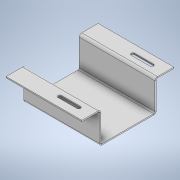
# Autodesk Inventor part: CameraProtection
Saved by Autodesk Inventor 2020 (Build 240168000, 168)
## iProperties
Created: 2019-11-07
Part Number: CameraProtection
Material: Generic
Document SubType Name: Sheet Metal
Designer: nicoc
Density: 1 g/cm^3
Sheet Metal Rule: Default_mm
Appearance: Default
Author: nicoc
Autodesk Inventor part; units mm, degrees
ref_plane "YZ Plane" through (0, 0, 0) normal (1, 0, 0) x (0, 1, 0)
ref_plane "XZ Plane" through (0, 0, 0) normal (0, 1, 0) x (-1, 0, 0)
ref_plane "XY Plane" through (0, 0, 0) normal (0, 0, 1) x (1, 0, 0)
sketch "Sketch1" plane through (0, 0, 0) normal (0, 1, 0) x (-1, 0, 0)
  line L0 (0, 0) -> (120, 0)
  line L1 (120, 0) -> (120, -30)
  line L2 (120, -30) -> (0, -30)
  line L3 (0, -30) -> (0, 0)
  dimension "d41" = 120
  dimension "d42" = 30
  measures "d41" distance between parallel lines of L1 L3
  measures "d42" distance between parallel lines of L0 L2
extrude "Plate1" add sketch "Sketch1" along normal mid plane 2
sketch "Sketch6" plane through (0, 1, -28) normal (0, 0, -1) x (-1, 0, 0)
  line L0 (120, 0) -> (0, 0)
  line L1 (0, 0) -> (0, -50)
  line L2 (0, -50) -> (120, -50)
  line L3 (120, -50) -> (120, 0)
  constraints: 6 end point, 1 horizontal, 1 perpendicular, 1 vertical
edge flange "Flange5" height 50 angle 90 thickness 2 bend radius 2 thickness toward (0, 0, -1) relief tear relief width 2 relief depth 1 edges at (-60, -1, -30) wall of the first edge with corners at (-120, 1, -28) (0, 1, -28) (0, -49, -28) (-120, -49, -28)
bend "Bend5"
corner "Corner5"
sketch "Sketch7" plane through (-120, -47, -28) normal (0, -1, 0) x (1, 0, 0)
  line L0 (120, 0) -> (0, 0)
  line L1 (0, 0) -> (0, -90)
  line L2 (0, -90) -> (120, -90)
  line L3 (120, -90) -> (120, 0)
  constraints: 6 end point, 1 horizontal, 1 perpendicular, 1 vertical
edge flange "Flange6" height 90 angle 90 thickness 2 bend radius 2 thickness toward (0, -1, 0) relief tear relief width 2 relief depth 1 edges at (-60, -49, -30) wall of the first edge with corners at (0, -47, -28) (-120, -47, -28) (-120, -47, -118) (0, -47, -118)
bend "Bend6"
corner "Corner6"
sketch "Sketch8" plane through (-120, -49, -116) normal (0, 0, -1) x (-1, 0, 0)
  line L0 (-120, 0) -> (0, 0)
  line L1 (0, 0) -> (0, 50)
  line L2 (0, 50) -> (-120, 50)
  line L3 (-120, 50) -> (-120, 0)
  constraints: 6 end point, 1 horizontal, 1 perpendicular, 1 vertical
edge flange "Flange7" height 50 angle 90 thickness 2 bend radius 2 thickness toward (0, 0, -1) relief tear relief width 2 relief depth 1 edges at (-60, -47, -118) wall of the first edge with corners at (0, -49, -116) (-120, -49, -116) (-120, 1, -116) (0, 1, -116)
bend "Bend7"
corner "Corner7"
sketch "Sketch9" plane through (0, -1, -116) normal (0, 1, 0) x (-1, 0, 0)
  line L0 (120, 0) -> (0, 0)
  line L1 (0, 0) -> (0, -30)
  line L2 (0, -30) -> (120, -30)
  line L3 (120, -30) -> (120, 0)
  constraints: 6 end point, 1 horizontal, 1 perpendicular, 1 vertical
edge flange "Flange8" height 30 angle 90 thickness 2 bend radius 2 thickness toward (0, 1, 0) relief tear relief width 2 relief depth 1 edges at (-60, 1, -118) wall of the first edge with corners at (-120, -1, -116) (0, -1, -116) (0, -1, -146) (-120, -1, -146)
bend "Bend8"
corner "Corner8"
sketch "Sketch15" plane through (0, -1, 0) normal (0, -1, 0) x (1, 0, 0)
  line L0 (-17.25, -15) -> (-52.75, -15) construction
  line L1 (-20, -17.75) -> (-50, -17.75)
  line L2 (-50, -12.25) -> (-20, -12.25)
  arc A0 (-20, -17.75) -> (-20, -12.25) centre (-20, -15) ccw
  arc A1 (-50, -12.25) -> (-50, -17.75) centre (-50, -15) ccw
  line L3 (0, -26) -> (0, 0) projected
  line L4 (0, 0) -> (-120, 0) projected
  point P0 (-35, -15)
  dimension "d130" = 20
  dimension "d131" = 15
  dimension "d132" = 30
  dimension "d133" = 5.5
  constraints: 8 end point, 6 point on circle, 4 tangent, 2 centre point, 2 point on line, 1 horizontal, 1 midpoint, 1 parallel
  measures "d130" distance from line of L3 A0.centre
  measures "d131" distance from line of L4 A0.centre
  measures "d132" distance of A1.centre A0.centre
  measures "d133" distance between parallel lines of L1 L2
extrude "Cut3" cut sketch "Sketch15" against normal blind 2
sketch "Sketch16" plane through (-120, -1, -146) normal (0, -1, 0) x (1, 0, 0)
  line L0 (102.75, 15) -> (67.25, 15) construction
  line L1 (100, 17.75) -> (70, 17.75)
  line L2 (70, 12.25) -> (100, 12.25)
  arc A0 (100, 12.25) -> (100, 17.75) centre (100, 15) ccw
  arc A1 (70, 17.75) -> (70, 12.25) centre (70, 15) ccw
  line L3 (120, 26) -> (120, 0) projected
  line L4 (0, 0) -> (120, 0) projected
  point P0 (120, 146)
  point P1 (85, 15)
  dimension "d136" = 20
  dimension "d137" = 15
  dimension "d138" = 5.5
  dimension "d139" = 30
  constraints: 8 end point, 6 point on circle, 4 tangent, 2 centre point, 2 point on line, 1 horizontal, 1 midpoint, 1 parallel
  measures "d136" distance from line of L3 A0.centre
  measures "d137" distance from line of L4 A0.centre
  measures "d138" distance between parallel lines of L2 L1
  measures "d139" distance of A1.centre A0.centre
extrude "Cut4" cut sketch "Sketch16" against normal blind 2
equation "\"d134\" = Thickness"
equation "\"d140\" = Thickness"
equation "\"d0\" = Thickness"
equation "\"d43\" = BendReliefWidth"
equation "\"d44\" = BendReliefDepth"
equation "\"d45\" = MinimumRemnant"
equation "\"d46\" = TransitionRadius"
equation "\"d49\" = BendRadius"
equation "\"d50\" = CornerReliefSize"
equation "\"d51\" = GapSize"
equation "\"d52\" = JacobiRadiusSize"
equation "\"d53\" = BendReliefWidth"
equation "\"d54\" = BendReliefDepth"
equation "\"d55\" = MinimumRemnant"
equation "\"d56\" = TransitionRadius"
equation "\"d59\" = BendRadius"
equation "\"d60\" = CornerReliefSize"
equation "\"d61\" = GapSize"
equation "\"d62\" = JacobiRadiusSize"
equation "\"d63\" = BendReliefWidth"
equation "\"d64\" = BendReliefDepth"
equation "\"d65\" = MinimumRemnant"
equation "\"d66\" = TransitionRadius"
equation "\"d69\" = BendRadius"
equation "\"d70\" = CornerReliefSize"
equation "\"d71\" = GapSize"
equation "\"d72\" = JacobiRadiusSize"
equation "\"d73\" = BendReliefWidth"
equation "\"d74\" = BendReliefDepth"
equation "\"d75\" = MinimumRemnant"
equation "\"d76\" = TransitionRadius"
equation "\"d79\" = BendRadius"
equation "\"d80\" = CornerReliefSize"
equation "\"d81\" = GapSize"
equation "\"d82\" = JacobiRadiusSize"
equation "\"BendRadius\" = Thickness"
equation "\"BendReliefWidth\" = Thickness"
equation "\"BendReliefDepth\" = 0.5 * Thickness"
equation "\"CornerReliefSize\" = 4 * Thickness"
equation "\"MinimumRemnant\" = 2 * Thickness"
equation "\"TransitionRadius\" = BendRadius"
equation "\"JacobiRadiusSize\" = BendRadius"
equation "\"GapSize\" = Thickness"
equation "\"Thickness\" = 2"
body "Solid1"
